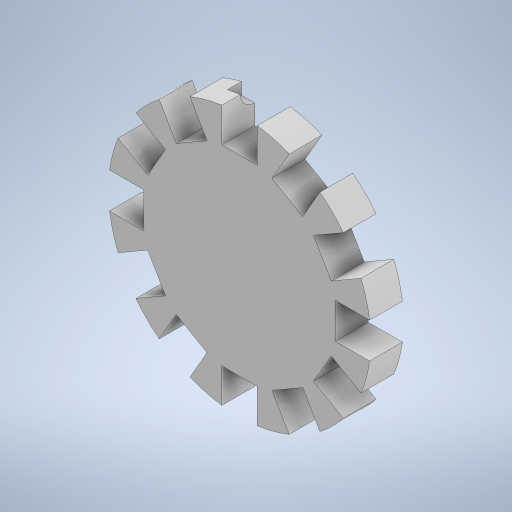
# Autodesk Inventor part: frame
Saved by Autodesk Inventor 2024.1 (Build 281209000, 209)
## iProperties
Created: 2024-06-29
Part Number: frame
Material: 一般
Document SubType Name: Modeling
Designer: hibik
Density: 1 g/cm^3
Appearance: 既定
Author: hibik
Autodesk Inventor part; units mm, degrees
ref_plane "YZ Plane" through (0, 0, 0) normal (1, 0, 0) x (0, 1, 0)
ref_plane "XZ Plane" through (0, 0, 0) normal (0, 1, 0) x (-1, 0, 0)
ref_plane "XY Plane" through (0, 0, 0) normal (0, 0, 1) x (1, 0, 0)
sketch "スケッチ1" plane through (0, 0, 0) normal (0, 0, 1) x (1, 0, 0)
  circle A0 centre (0, 0) radius 10
  line L0 (-1.35, 10) -> (1.35, 10) construction
  line L1 (1.35, 10) -> (1.35, 7.3)
  line L2 (1.35, 7.3) -> (-1.35, 7.3)
  line L3 (-1.35, 7.3) -> (-1.35, 10)
  line L4 (-4.8191, 5.647) -> (-6.1691, 7.9853)
  line L5 (-3.8309, 9.3353) -> (-2.4809, 6.997)
  line L6 (-2.4809, 6.997) -> (-4.8191, 5.647)
  line L7 (-6.997, 2.4809) -> (-9.3353, 3.8309)
  line L8 (-7.9853, 6.1691) -> (-5.647, 4.8191)
  line L9 (-5.647, 4.8191) -> (-6.997, 2.4809)
  line L10 (-7.3, -1.35) -> (-10, -1.35)
  line L11 (-10, 1.35) -> (-7.3, 1.35)
  line L12 (-7.3, 1.35) -> (-7.3, -1.35)
  line L13 (-5.647, -4.8191) -> (-7.9853, -6.1691)
  line L14 (-9.3353, -3.8309) -> (-6.997, -2.4809)
  line L15 (-6.997, -2.4809) -> (-5.647, -4.8191)
  line L16 (-2.4809, -6.997) -> (-3.8309, -9.3353)
  line L17 (-6.1691, -7.9853) -> (-4.8191, -5.647)
  line L18 (-4.8191, -5.647) -> (-2.4809, -6.997)
  line L19 (1.35, -7.3) -> (1.35, -10)
  line L20 (-1.35, -10) -> (-1.35, -7.3)
  line L21 (-1.35, -7.3) -> (1.35, -7.3)
  line L22 (4.8191, -5.647) -> (6.1691, -7.9853)
  line L23 (3.8309, -9.3353) -> (2.4809, -6.997)
  line L24 (2.4809, -6.997) -> (4.8191, -5.647)
  line L25 (6.997, -2.4809) -> (9.3353, -3.8309)
  line L26 (7.9853, -6.1691) -> (5.647, -4.8191)
  line L27 (5.647, -4.8191) -> (6.997, -2.4809)
  line L28 (7.3, 1.35) -> (10, 1.35)
  line L29 (10, -1.35) -> (7.3, -1.35)
  line L30 (7.3, -1.35) -> (7.3, 1.35)
  line L31 (5.647, 4.8191) -> (7.9853, 6.1691)
  line L32 (9.3353, 3.8309) -> (6.997, 2.4809)
  line L33 (6.997, 2.4809) -> (5.647, 4.8191)
  line L34 (2.4809, 6.997) -> (3.8309, 9.3353)
  line L35 (6.1691, 7.9853) -> (4.8191, 5.647)
  line L36 (4.8191, 5.647) -> (2.4809, 6.997)
  point P0 (0, 10)
  point P1 (-1.35, 9.9085)
  point P2 (-3.7851, 9.256)
  point P3 (-6.1234, 7.906)
  point P4 (-7.906, 6.1234)
  point P5 (-9.256, 3.7851)
  point P6 (-9.9085, 1.35)
  point P7 (-9.9085, -1.35)
  point P8 (-9.256, -3.7851)
  point P9 (-7.906, -6.1234)
  point P10 (-6.1234, -7.906)
  point P11 (-3.7851, -9.256)
  point P12 (-1.35, -9.9085)
  point P13 (1.35, -9.9085)
  point P14 (3.7851, -9.256)
  point P15 (6.1234, -7.906)
  point P16 (7.906, -6.1234)
  point P17 (9.256, -3.7851)
  point P18 (9.9085, -1.35)
  point P19 (9.9085, 1.35)
  point P20 (9.256, 3.7851)
  point P21 (7.906, 6.1234)
  point P22 (6.1234, 7.906)
  point P23 (3.7851, 9.256)
  point P24 (1.35, 9.9085)
  dimension "d0" = 20
  dimension "d3" = 2.7
  dimension "d4" = 2.7
  dimension "d7" = 360
  constraints: 74 end point, 2 horizontal, 2 parallel, 1 coincident, 1 midpoint, 1 perpendicular, 1 vertical alignment, 87 other
  measures "d3" distance of L1.end L2.end
  measures "d4" distance of L0.end L1.end
extrude "押し出し2" add sketch "スケッチ1" along normal blind 2.5 contours L28 L30 L29 A0 L25 L27 L26 L22 L24 L23 L19 L21 L20 L16 L18 L17 L13 L15 L14 L10 L12 L11 L7 L9 L8 L4 L6 L5 L3 L2 L1 L34 L36 L35 L31 L33 L32
sketch "スケッチ2" plane through (-1.35, 7.3, 0) normal (1, 0, 0) x (0, 0, -1)
  line L0 (0, 0) -> (0, 2.6085) projected
  circle A0 centre (0, 2.6085) radius 1.1
  point P0 (0, -7.3)
  dimension "d11" = 2.2
  constraints: 1 centre point
  measures "d11" diameter of A0
extrude "押し出し3" cut sketch "スケッチ2" against normal blind 1
